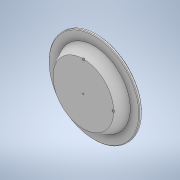
# Autodesk Inventor part: printingPlatform
Saved by Autodesk Inventor 2020 (Build 240168000, 168)
## iProperties
Created: 2020-03-25
Part Number: printingPlatform
Material: Generic
Document SubType Name: Modeling
Designer: zhang
Density: 1 g/cm^3
Appearance: Default
Author: zhang
Autodesk Inventor part; units mm, degrees
ref_plane "YZ Plane" through (0, 0, 0) normal (1, 0, 0) x (0, 1, 0)
ref_plane "XZ Plane" through (0, 0, 0) normal (0, 1, 0) x (-1, 0, 0)
ref_plane "XY Plane" through (0, 0, 0) normal (0, 0, 1) x (1, 0, 0)
sketch "Sketch1" plane through (0, 0, 0) normal (0, 0, 1) x (1, 0, 0)
  circle A0 centre (0, 0) radius 150
  dimension "d0" = 300
  constraints: 1 centre point, 1 coincident
  measures "d0" diameter of A0
extrude "Extrusion1" add sketch "Sketch1" against normal blind 4
sketch "Sketch5" plane through (0, 0, 0) normal (0, 1, 0) x (-1, 0, 0)
  line L0 (150, 0) -> (-150, 0) projected
  line L1 (100, 40) -> (0, 40)
  line L2 (0, 40) -> (0, 0)
  line L3 (-150, -4) -> (150, -4) projected
  line L4 (150, 0) -> (0, 0)
  line L5 (100, 40) -> (120, 5)
  line L6 (120, 5) -> (150, 5)
  line L7 (150, 0) -> (150, 5)
  dimension "d16" = 40
  dimension "d17" = 100
  dimension "d21" = 30
  dimension "d22" = 5
  constraints: 12 end point, 2 perpendicular, 1 horizontal, 1 parallel, 1 vertical
  measures "d16" distance of L1.end L2.end
  measures "d17" distance of L1.start L1.end
  measures "d21" distance of L5.end L6.end
  measures "d22" distance of L0.start L6.end
revolve "Revolution2" add sketch "Sketch5" angle 360 about axis through (0, 0, 40) along (0, 0, -1)
shell "Shell1" thickness 10 removed faces 1 at (43.9875, -8.828, -4)
chamfer "Chamfer2" distance 2 angle 45 3 edges at (0, 150, -4) (0, -150, -4) (150, 0, 5)
chamfer "Chamfer3" distance 2 angle 45 2 edges at (113.6253, 0.004, -4) (94.1968, 0, 30)
sketch "Sketch7" plane through (0, 0, 40) normal (0, 0, 1) x (1, 0, 0)
  line L0 (-3.0843, 115) -> (2.9157, 115)
  line L1 (2.9157, 115) -> (2.9157, 95)
  line L2 (2.9157, 95) -> (-3.0843, 95)
  line L3 (-3.0843, 95) -> (-3.0843, 115)
  line L4 (0, 122.9012) -> (0, 72.4228)
  line L5 (95, 3.0843) -> (115, 3.0843)
  line L6 (115, 3.0843) -> (115, -2.9157)
  line L7 (115, -2.9157) -> (95, -2.9157)
  line L8 (95, -2.9157) -> (95, 3.0843)
  circle A0 centre (0, 0) radius 2
  dimension "d33" = 6
  dimension "d34" = 20
  dimension "d35" = 95
  dimension "d38" = 90
  dimension "d42" = 4
  constraints: 18 end point, 2 parallel, 2 vertical, 1 centre point, 1 coincident, 1 horizontal, 1 perpendicular, 9 other
  measures "d33" distance of L1.end L2.end
  measures "d34" distance of L0.end L1.end
  measures "d35" distance from line of point (0, 0) L2
  measures "d42" diameter of A0
extrude "Extrusion4" cut sketch "Sketch7" against normal blind 2
body "Solid1"
